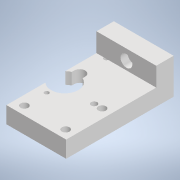
# Autodesk Inventor part: Hand1
Saved by Autodesk Inventor 2022 (Build 260153000, 153)
## iProperties
Created: 2021-06-22
Part Number: Hand1
Material: Generic
Document SubType Name: Modeling
Designer: Prajwal Patil
Density: 1 g/cm^3
Appearance: Default
Author: Prajwal Patil
Autodesk Inventor part; units mm, degrees
ref_plane "YZ Plane" through (0, 0, 0) normal (1, 0, 0) x (0, 1, 0)
ref_plane "XZ Plane" through (0, 0, 0) normal (0, 1, 0) x (-1, 0, 0)
sketch "Sketch1" plane through (0, 0, 0) normal (0, 1, 0) x (-1, 0, 0)
  line L0 (17.0879, 31.457) -> (-17.8371, 31.457)
  line L1 (-17.8371, 31.457) -> (-17.8371, -31.3318)
  line L2 (-17.8371, -31.3318) -> (17.0879, -31.3318)
  line L3 (17.0879, -31.3318) -> (17.0879, 31.457)
  point P0 (0, 0)
  dimension "d0" = 34.925
  dimension "d1" = 62.7888
  constraints: 8 end point, 2 parallel, 1 horizontal, 1 perpendicular
  measures "d0" distance of L2.end L1.end
  measures "d1" distance of L1.end L0.end
extrude "Extrusion1" add sketch "Sketch1" along normal blind 9.7028
sketch "Sketch2" plane through (0, 9.7028, 0) normal (0, 1, 0) x (1, 0, 0)
  line L0 (17.8371, -31.457) -> (17.8371, 31.3318) projected
  line L1 (-17.0879, 31.3318) -> (-17.0879, -31.457) projected
  line L2 (17.8371, 31.3318) -> (-17.0879, 31.3318)
  line L3 (-17.0879, 31.3318) -> (-17.0879, 21.1718)
  line L4 (-17.0879, 21.1718) -> (17.8371, 21.1718)
  line L5 (17.8371, 21.1718) -> (17.8371, 31.3318)
  point P0 (0, 0)
  dimension "d4" = 10.16
  constraints: 8 end point, 2 parallel, 1 horizontal, 1 perpendicular, 1 point on line
  measures "d4" distance of L3.end L2.end
extrude "Extrusion2" add sketch "Sketch2" along normal blind 11.049
sketch "Sketch3" plane through (0, 0, 0) normal (0, -1, 0) x (1, 0, 0)
  line L0 (17.8371, -31.3318) -> (-17.0879, -31.3318) projected
  line L1 (-17.0879, -31.3318) -> (-17.0879, -25.0072)
  line L2 (-17.0879, -31.3318) -> (-17.0879, 31.457) projected
  line L3 (-17.0879, -25.0072) -> (-3.5751, -25.0072)
  line L4 (-3.5751, -25.0072) -> (-3.5751, -18.962)
  line L5 (-3.5751, -18.962) -> (-3.2703, -18.962)
  line L6 (-3.2703, -18.962) -> (-3.2703, 10.883)
  line L7 (-3.2703, 10.883) -> (-3.5751, 10.883)
  line L8 (-3.5751, 10.883) -> (-3.5751, 16.9282)
  line L9 (-3.5751, 16.9282) -> (-16.9609, 16.9282)
  line L10 (-16.9609, 16.9282) -> (-17.0879, 16.9282)
  point P0 (0, 0)
  dimension "d7" = 6.3246
  dimension "d8" = 13.5128
  dimension "d9" = 6.0452
  dimension "d10" = 0.3048
  dimension "d11" = 29.845
  dimension "d14" = 0.3048
  dimension "d15" = 6.0452
  dimension "d16" = 13.3858
  constraints: 18 end point, 5 perpendicular, 3 point on line, 2 horizontal
  measures "d7" distance of L0.end L1.end
  measures "d8" distance of L1.end L3.end
  measures "d9" distance of L3.end L4.end
  measures "d10" distance of L4.end L5.end
  measures "d11" distance of L5.end L6.end
  measures "d14" distance of L6.end L7.end
  measures "d15" distance of L7.end L8.end
  measures "d16" distance of L8.end L9.end
extrude "Extrusion3" cut sketch "Sketch3" against normal blind 2.794
sketch "Sketch4" plane through (0, 2.794, 0) normal (0, -1, 0) x (1, 0, 0)
  line L0 (-3.5751, 16.9282) -> (-17.0879, 16.9282)
  line L1 (-17.0879, 16.9282) -> (-17.0879, 10.883)
  line L2 (-17.0879, 10.883) -> (-3.5751, 10.883)
  line L3 (-3.5751, 10.883) -> (-3.5751, 16.9282)
  point P0 (0, 0)
  dimension "d19" = 13.5128
  dimension "d20" = 6.0452
  constraints: 8 end point, 2 parallel, 1 horizontal, 1 perpendicular
  measures "d19" distance of L2.end L1.end
  measures "d20" distance of L1.end L0.end
sketch "Sketch5" plane through (0, 2.794, 0) normal (0, -1, 0) x (1, 0, 0)
  line L0 (-3.5751, -18.962) -> (-3.5751, -25.0072) projected
  line L1 (-3.5751, -25.0072) -> (-17.0879, -25.0072)
  line L2 (-17.0879, -25.0072) -> (-17.0879, -18.962)
  line L3 (-17.0879, -18.962) -> (-3.5751, -18.962)
  line L4 (-3.5751, -18.962) -> (-3.5751, -25.0072)
  point P0 (0, 0)
  dimension "d21" = 13.5128
  dimension "d22" = 6.0452
  constraints: 8 end point, 2 parallel, 1 horizontal, 1 perpendicular
  measures "d21" distance of L2.end L3.end
  measures "d22" distance of L1.end L2.end
extrude "Extrusion5" add sketch "Sketch4" along normal blind 1.5748
extrude "Extrusion6" add sketch "Sketch5" along normal blind 1.5748
sketch "Sketch6" plane through (0, 9.7028, 0) normal (0, 1, 0) x (1, 0, 0)
  circle A0 centre (-11.6221, -2.8625) radius 7.9629
  line L0 (-17.0879, 18.962) -> (-17.0879, -10.883) projected
  line L1 (-11.6221, -10.1806) -> (-11.6221, 5.913) construction
  line L2 (-14.7946, -10.1806) -> (-14.7946, 5.913)
  line L3 (-8.4496, 5.913) -> (-8.4496, -10.1806)
  arc A1 (-8.4496, 5.913) -> (-14.7946, 5.913) centre (-11.6221, 5.913) ccw
  point P0 (0, 0)
  point P1 (-17.0879, 21.1718)
  point P2 (-11.6221, -2.1338)
  point P3 (-17.0879, 2.9283)
  point P4 (-17.0879, -8.6532)
  point P5 (-8.4496, 4.4412)
  point P6 (-14.7946, 4.4412)
  dimension "d31" = 15.9258
  constraints: 8 end point, 2 centre point, 2 point on circle, 2 tangent, 1 midpoint, 1 parallel, 1 point on line
  measures "d31" diameter of A0
extrude "Extrusion7" cut sketch "Sketch6" against normal blind 25.4 contours A0 L3 | L3 A0 L2 | A0 L2 A1 L3 | L2 A0 L0
ref_plane "Work Plane1" through (0, 0, 0) normal (0, 1, 0) x (1, 0, 0)
sketch "Sketch7" plane through (0, 9.7028, 0) normal (0, 1, 0) x (1, 0, 0)
  line L0 (17.8371, -31.457) -> (17.8371, -28.663)
  line L1 (17.8371, -28.663) -> (17.8371, -26.4532)
  line L2 (14.7637, -26.4532) -> (12.5539, -26.4532)
  circle A0 centre (12.5539, -26.4532) radius 2.2098
  circle A1 centre (12.5539, -5.168) radius 2.2098
  line L3 (-17.0879, -8.6532) -> (-17.0879, -31.457) projected
  line L4 (-17.0879, -26.4532) -> (-13.7859, -26.4532) construction
  circle A2 centre (-11.5761, -26.4532) radius 2.2098
  line L5 (-11.5761, -14.7184) -> (-11.5761, -13.4484)
  circle A3 centre (-11.5761, -13.4484) radius 1.27
  line L6 (-11.5761, -13.4484) -> (-17.0879, -13.4484)
  line L7 (-17.0879, -16.9282) -> (-17.0879, -10.883) projected
  circle A4 centre (12.5539, -5.168) radius 4.1148
  circle A5 centre (12.5539, -26.4532) radius 4.1148
  circle A6 centre (-11.5761, -26.4532) radius 4.1148
  point P0 (0, 0)
  dimension "d37" = 2.794
  dimension "d38" = 2.2098
  dimension "d39" = 3.0734
  dimension "d40" = 2.2098
  dimension "d42" = 4.4196
  dimension "d43" = 4.4196
  dimension "d47" = 4.4196
  dimension "d49" = 1.27
  dimension "d50" = 2.54
  dimension "d58" = 8.2296
  dimension "d59" = 8.2296
  dimension "d60" = 8.2296
  constraints: 12 end point, 7 centre point, 5 coincident, 3 point on line, 1 horizontal, 1 perpendicular
  measures "d37" distance of L0.start L0.end
  measures "d38" distance of L0.end L1.end
  measures "d39" distance of L1.end L2.start
  measures "d40" distance of L2.start L2.end
  measures "d42" diameter of A0
  measures "d43" diameter of A1
  measures "d47" diameter of A2
  measures "d49" distance of L5.start L5.end
  measures "d50" diameter of A3
  measures "d58" diameter of A4
  measures "d59" diameter of A5
  measures "d60" diameter of A6
extrude "Extrusion8" cut sketch "Sketch7" against normal blind 25.4 contours A0 | A1 | A2 | A3 L6 L5 | L5 L6 A3
sketch "Sketch9" plane through (0, 1.2192, 0) normal (0, -1, 0) x (1, 0, 0)
  line L0 (-3.5751, -18.962) -> (-17.0879, -18.962) projected
  line L1 (-17.0879, -18.962) -> (-11.5761, -18.962)
  line L2 (-11.5761, -25.0595) -> (-11.5761, -21.2495)
  circle A0 centre (-11.5761, -21.2495) radius 1.27
  point P0 (0, 0)
  dimension "d53" = 5.5118
  dimension "d54" = 3.81
  dimension "d55" = 2.54
  constraints: 4 end point, 1 centre point, 1 coincident, 1 point on line
  measures "d53" distance of L0.end L1.end
  measures "d54" distance of L2.start L2.end
  measures "d55" diameter of A0
extrude "Extrusion9" cut sketch "Sketch9" against normal blind 8.4836
sketch "Sketch11" plane through (0, 0, 0) normal (0, -1, 0) x (1, 0, 0)
  circle A0 centre (-11.5761, 26.4532) radius 2.2098 projected
  circle A1 centre (-11.5761, 26.4532) radius 4.1148
  circle A2 centre (12.5539, 26.4532) radius 2.2098 projected
  circle A3 centre (12.5539, 26.4532) radius 4.1148
  circle A4 centre (12.5539, 5.168) radius 2.2098 projected
  circle A5 centre (12.5539, 5.168) radius 4.1148
  point P0 (0, 0)
  dimension "d62" = 8.2296
  dimension "d63" = 8.2296
  dimension "d64" = 8.2296
  constraints: 3 centre point, 3 coincident
  measures "d62" diameter of A1
  measures "d63" diameter of A3
  measures "d64" diameter of A5
extrude "Extrusion10" cut sketch "Sketch11" against normal blind 5.6642 contours A0 | A1 | A3 | A5
sketch "Sketch12" plane through (17.8371, 0, -31.3318) normal (0, 0, -1) x (-1, 0, 0)
  line L0 (0, 0) -> (0, 20.7518) projected
  line L1 (0, 20.7518) -> (13.9446, 20.7518)
  line L2 (0, 20.7518) -> (34.925, 20.7518) projected
  line L3 (13.9446, 20.7518) -> (17.4117, 20.7518)
  line L4 (17.4117, 20.7518) -> (17.4117, 17.9832)
  line L5 (17.4117, 17.9832) -> (17.4117, 14.5161)
  circle A0 centre (17.4117, 14.5161) radius 2.2479
  circle A1 centre (17.4117, 14.5161) radius 3.4671
  point P0 (17.8371, 0)
  dimension "d67" = 13.9446
  dimension "d68" = 3.4671
  dimension "d69" = 2.7686
  dimension "d70" = 3.4671
  dimension "d71" = 4.4958
  dimension "d72" = 6.9342
  constraints: 8 end point, 3 point on line, 2 centre point, 2 coincident, 1 perpendicular
  measures "d67" distance of L0.end L1.end
  measures "d68" distance of L1.end L3.end
  measures "d69" distance of L3.end L4.end
  measures "d70" distance of L4.end L5.end
  measures "d71" diameter of A0
  measures "d72" diameter of A1
extrude "Extrusion11" cut sketch "Sketch12" against normal through all contours A0
extrude "Extrusion13" cut sketch "Sketch12" against normal blind 4.4958
sketch "Sketch13" plane through (-17.0879, 20.7518, -21.1718) normal (0, 0, 1) x (1, 0, 0)
  circle A0 centre (17.5133, -6.2357) radius 3.4671 projected
  circle A1 centre (17.5133, -6.2357) radius 2.7813
  point P0 (17.0879, -20.7518)
  dimension "d79" = 5.5626
  constraints: 1 centre point, 1 coincident
  measures "d79" diameter of A1
extrude "Extrusion14" cut sketch "Sketch13" against normal blind 4.1656 contours A0 | A1
sketch "Sketch14" plane through (0, 9.7028, 0) normal (0, 1, 0) x (1, 0, 0)
  circle A0 centre (7.9099, -5.168) radius 1.7354
  point P0 (0, 0)
  constraints: 1 centre point
extrude "Extrusion15" cut sketch "Sketch14" against normal blind 12.7
body "Solid1"
